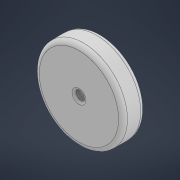
# Autodesk Inventor part: roller
Saved by Autodesk Inventor 2022 (Build 260153000, 153)
## iProperties
Created: 2024-10-24
Part Number: roller
Material: Generic
Document SubType Name: Modeling
Designer: HCI
Density: 1 g/cm^3
Appearance: Default
Author: HCI
Autodesk Inventor part; units mm, degrees
ref_plane "YZ Plane" through (0, 0, 0) normal (1, 0, 0) x (0, 1, 0)
ref_plane "XZ Plane" through (0, 0, 0) normal (0, 1, 0) x (-1, 0, 0)
ref_plane "XY Plane" through (0, 0, 0) normal (0, 0, 1) x (1, 0, 0)
sketch "Sketch1" plane through (0, 0, 0) normal (0, 0, 1) x (1, 0, 0)
  circle A0 centre (0, 0) radius 2.15
  circle A1 centre (0, 0) radius 20
  dimension "d0" = 4.3
  dimension "d1" = 40
  constraints: 2 centre point, 2 coincident
  measures "d0" diameter of A0
  measures "d1" diameter of A1
extrude "Extrusion1" add sketch "Sketch1" along normal blind 10
fillet "Fillet1" radius 2 2 edges at (-20, 0, 10) (-20, 0, 0)
fillet "Fillet2" radius 1 2 edges at (-2.15, 0, 10) (-2.15, 0, 0)
body "Solid1"
